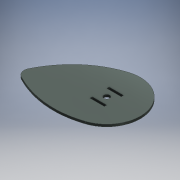
# Autodesk Inventor part: leva00
Saved by Autodesk Inventor 2016 (Build 200138000, 138)
## iProperties
Created: 2016-09-20
Part Number: leva00
Material: Madera (abedul)
Document SubType Name: Modeling
Designer: i95sa
Density: 0.55 g/cm^3
Appearance: Gris plomo - Pulido
Author: i95sa
Autodesk Inventor part; units mm, degrees
ref_plane "YZ Plane" through (0, 0, 0) normal (1, 0, 0) x (0, 1, 0)
ref_plane "XZ Plane" through (0, 0, 0) normal (0, 1, 0) x (-1, 0, 0)
ref_plane "XY Plane" through (0, 0, 0) normal (0, 0, 1) x (1, 0, 0)
sketch "Boceto1" plane through (0, 0, 0) normal (0, 0, 1) x (1, 0, 0)
  arc A0 (55.3277, 17.9771) -> (-55.3277, -17.9771) centre (0, 0) ccw
  arc A1 (-85.145, -27.6653) -> (-110.6809, -35.9624) centre (-97.9129, -31.8138) ccw
  line L0 (-114.3775, -37.1635) -> (-118.5261, -24.3956)
  line L1 (-17.3204, 55.5368) -> (-24.2347, 76.8167)
  line L2 (-24.2347, 76.8167) -> (-118.5261, -24.3956)
  line L3 (-118.5261, -24.3956) -> (-81.9216, 14.8956)
  arc A2 (-17.3204, 55.5368) -> (-81.9216, 14.8956) centre (27.0018, -86.5796) ccw
  arc A3 (-81.9216, 14.8956) -> (-109.9762, -25.9225) centre (41.0775, -99.6928) ccw
  line L4 (4.256, 1.3829) -> (55.3277, 17.9771)
  line L5 (-4.256, -1.3829) -> (-114.3775, -37.1635)
  arc A4 (-55.3277, -17.9771) -> (55.3277, 17.9771) centre (0, 0) ccw
  arc A5 (-110.6809, -35.9624) -> (-85.145, -27.6653) centre (-97.9129, -31.8138) ccw
  line L6 (-114.3775, -37.1635) -> (-110.229, -49.9314)
  line L7 (18.6312, -55.1109) -> (25.5455, -76.3908)
  line L8 (25.5455, -76.3908) -> (-110.229, -49.9314)
  line L9 (-110.229, -49.9314) -> (-57.5205, -60.2031)
  arc A6 (-57.5205, -60.2031) -> (18.6312, -55.1109) centre (-29.0453, 85.9156) ccw
  arc A7 (-104.2095, -43.6707) -> (-57.5205, -60.2031) centre (-25.3655, 104.798) ccw
  dimension "d0" = 116.35
  dimension "d6" = 26.85
  dimension "d7" = 13.425
  dimension "d8" = 22.375
  dimension "d9" = 53.7
  constraints: 20 end point, 20 point on circle, 8 centre point, 6 symmetric about line, 5 point on line, 4 tangent, 1 collinear, 4 other
  measures "d0" diameter of A0
  measures "d6" diameter of A1
  measures "d7" distance of L0.start L0.end
  measures "d8" distance of L1.start L1.end
  measures "d9" distance of L0.end L3.end
extrude "Extrusión2" add sketch "Boceto1" along normal blind 4 contours A4 A0 | A0 L5 A1 A3 A2 | A6 A7 A5 L5 A4 | L5 A1 | A5 L5
sketch "Boceto2" plane through (0, 0, 4) normal (0, 0, 1) x (1, 0, 0)
  line L0 (0, 0) -> (0, 12.5)
  line L1 (0, 12.5) -> (-12.5, 12.5)
  line L2 (-12.5, 12.5) -> (-12.5, 16.7)
  line L3 (-12.5, 16.7) -> (12.5, 16.7)
  line L4 (12.5, 16.7) -> (12.5, 12.5)
  line L5 (12.5, 12.5) -> (0, 12.5)
  line L6 (0, 0) -> (12.5, 0)
  line L7 (0, 0) -> (0, -12.5)
  line L8 (0, -12.5) -> (-12.5, -12.5)
  line L9 (-12.5, -12.5) -> (-12.5, -16.7)
  line L10 (-12.5, -16.7) -> (12.5, -16.7)
  line L11 (12.5, -16.7) -> (12.5, -12.5)
  line L12 (12.5, -12.5) -> (0, -12.5)
  circle A0 centre (0, 0) radius 5
  dimension "d24" = 12.5
  dimension "d25" = 12.5
  dimension "d26" = 4.2
  dimension "d27" = 25
  dimension "d28" = 10
  constraints: 26 end point, 5 perpendicular, 5 symmetric about line, 3 point on line, 1 centre point, 1 coincident, 1 parallel, 1 vertical
  measures "d24" distance of L0.start L0.end
  measures "d25" distance of L0.end L1.end
  measures "d26" distance of L1.end L2.end
  measures "d27" distance of L2.end L3.end
  measures "d28" diameter of A0
extrude "Extrusión3" cut sketch "Boceto2" against normal blind 4
